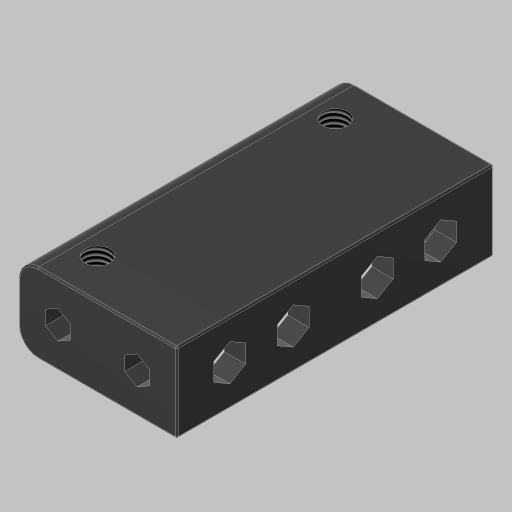
# Autodesk Inventor part: EL2-038
Saved by Autodesk Inventor 2023.5 (Build 275446000, 446)
## iProperties
Created: 2025-01-21
Part Number: EL2-038
Material: Thermoplastic Resin
Document SubType Name: Modeling
Designer: slick
Density: 1.28 g/cm^3
Appearance: Smooth - Black
Author: slick
Autodesk Inventor part; units mm, degrees
ref_plane "YZ Plane" through (0, 0, 0) normal (1, 0, 0) x (0, 1, 0)
ref_plane "XZ Plane" through (0, 0, 0) normal (0, 1, 0) x (-1, 0, 0)
ref_plane "XY Plane" through (0, 0, 0) normal (0, 0, 1) x (1, 0, 0)
sketch "Sketch1" plane through (0, 0, 0) normal (0, 0, 1) x (1, 0, 0)
  line L0 (-12.7, 6.35) -> (12.7, 6.35)
  line L1 (12.7, 6.35) -> (12.7, -6.35)
  line L2 (12.7, -6.35) -> (-12.7, -6.35)
  line L3 (-12.7, -6.35) -> (-12.7, 6.35)
  line L4 (-12.7, 6.35) -> (12.7, -6.35) construction
  line L5 (12.7, 6.35) -> (-12.7, -6.35) construction
  point P0 (0, 0)
  dimension "d0" = 25.4
  dimension "d1" = 12.7
  constraints: 12 end point, 2 midpoint, 2 parallel, 1 horizontal, 1 perpendicular
  measures "d0" distance of L1.end L2.end
  measures "d1" distance of L0.end L1.end
extrude "Extrusion1" add sketch "Sketch1" along normal mid plane 50.8
sketch "Sketch2" plane through (-12.7, 6.35, 25.4) normal (0, 1, 0) x (1, 0, 0)
  line L0 (6.35, 44.45) -> (6.35, 6.35) construction
  line L1 (0, 50.8) -> (0, 0) projected
  point P0 (12.7, 25.4)
  point P1 (6.35, 25.4)
  dimension "d4" = 38.1
  dimension "d5" = 6.35
  constraints: 2 end point, 1 horizontal alignment, 1 midpoint, 1 vertical, 1 vertical alignment
  measures "d4" distance of L0.start L0.end
  measures "d5" distance between parallel lines of L1 L0
hole "Hole1" at (-6.35, 6.35, 19.05) at (-6.35, 6.35, -19.05) direction (0, -1, 0) diameter 3.9624 end through all thread size "10-32 UNF" class "2B" standard "ANSI Unified Screw Threads"
fillet "Fillet1" radius 3.175 2 edges at (-12.7, 6.35, 0) (-12.7, -6.35, 0)
fillet "Fillet2" radius 0.254 14 edges at (-11.7701, 5.4201, 25.4) (-12.7, 0, 25.4) (-11.7701, -5.4201, 25.4) (1.5875, -6.35, 25.4) (1.5875, 6.35, 25.4) (12.7, 6.35, 0) (12.7, -6.35, 0) (12.7, 0, -25.4) (12.7, 0, 25.4) (-11.7701, 5.4201, -25.4) (-12.7, 0, -25.4) (-11.7701, -5.4201, -25.4) (1.5875, -6.35, -25.4) (1.5875, 6.35, -25.4)
sketch "Sketch3" plane through (-9.525, -6.35, 25.146) normal (0, -1, 0) x (1, 0, 0)
  line L0 (21.971, -50.292) -> (21.971, 0) projected
  line L1 (0, 0) -> (21.971, 0) projected
  line L2 (0, 0) -> (0, -50.292) projected
  line L3 (21.971, -50.292) -> (0, -50.292) projected
  circle A0 centre (3.175, -6.096) radius 1.9812 projected
  circle A1 centre (3.175, -44.196) radius 1.9812 projected
  line L4 (18.796, -3.175) -> (18.796, -47.117)
  line L5 (18.796, -47.117) -> (3.175, -47.117) construction
  line L6 (3.175, -47.117) -> (3.175, -3.175) construction
  line L7 (3.175, -3.175) -> (18.796, -3.175) construction
  circle A2 centre (3.175, -6.096) radius 5.1562 construction
  circle A3 centre (3.175, -44.196) radius 5.1562 construction
  line L8 (18.796, -3.175) -> (7.424, -3.175)
  line L9 (7.424, -47.117) -> (18.796, -47.117)
  arc A4 (0, -10.1587) -> (7.424, -3.175) centre (3.175, -6.096) ccw
  circle A5 centre (3.175, -44.196) radius 1.9812 projected
  arc A6 (7.424, -47.117) -> (0, -40.1333) centre (3.175, -44.196) ccw
  line L10 (21.971, -50.292) -> (21.971, 0) construction
  line L11 (0, 0) -> (21.971, 0) construction
  line L12 (0, 0) -> (0, -50.292) construction
  line L13 (21.971, -50.292) -> (0, -50.292) construction
  circle A7 centre (3.175, -6.096) radius 1.9812 construction
  circle A8 centre (3.175, -44.196) radius 1.9812 construction
  line L14 (0, 0) -> (0, -50.292) projected
  line L15 (0, -40.1333) -> (0, -10.1587)
  point P0 (9.525, -25.146)
  dimension "d15" = 3.175
  dimension "d16" = 3.175
  dimension "d17" = 3.175
  constraints: 14 end point, 8 point on circle, 4 centre point, 4 point on line, 2 coincident, 3 other
  measures "d15" distance between parallel lines of L0 L4
  measures "d16" radial gap between concentric circles of A0 A2
  measures "d17" radial gap between concentric circles of A1 A3
extrude "Extrusion2" cut sketch "Sketch3" against normal blind 9.525 contours L2 A4 L8 L4 L9 A6
fillet "Fillet3" radius 3.302 6 edges at (-2.101, -1.5875, 21.971) (9.271, -1.5875, 21.971) (9.271, -1.5875, -21.971) (-2.101, -1.5875, -21.971) (-9.525, -1.5875, -14.9873) (-9.525, -1.5875, 14.9873)
sketch "Sketch4" plane through (12.7, -6.096, 25.146) normal (1, 0, 0) x (0, 0, -1)
  line L0 (8.255, 9.0289) -> (10.795, 7.5625)
  line L1 (10.795, 7.5625) -> (10.795, 4.6295)
  line L2 (10.795, 4.6295) -> (8.255, 3.1631)
  line L3 (8.255, 3.1631) -> (5.715, 4.6295)
  line L4 (5.715, 4.6295) -> (5.715, 7.5625)
  line L5 (5.715, 7.5625) -> (8.255, 9.0289)
  line L6 (0, 0) -> (0, 12.192) construction
  line L7 (0, 12.192) -> (50.292, 12.192) construction
  line L8 (18.415, 9.0289) -> (20.955, 7.5625)
  line L9 (20.955, 7.5625) -> (20.955, 4.6295)
  line L10 (20.955, 4.6295) -> (18.415, 3.1631)
  line L11 (18.415, 3.1631) -> (15.875, 4.6295)
  line L12 (15.875, 4.6295) -> (15.875, 7.5625)
  line L13 (15.875, 7.5625) -> (18.415, 9.0289)
  line L14 (25.146, 12.192) -> (25.146, -0.254) construction
  line L15 (0, -0.254) -> (50.292, -0.254) construction
  line L16 (42.037, 9.0289) -> (39.497, 7.5625)
  line L17 (39.497, 7.5625) -> (39.497, 4.6295)
  line L18 (39.497, 4.6295) -> (42.037, 3.1631)
  line L19 (42.037, 3.1631) -> (44.577, 4.6295)
  line L20 (44.577, 4.6295) -> (44.577, 7.5625)
  line L21 (44.577, 7.5625) -> (42.037, 9.0289)
  line L22 (31.877, 9.0289) -> (29.337, 7.5625)
  line L23 (29.337, 7.5625) -> (29.337, 4.6295)
  line L24 (29.337, 4.6295) -> (31.877, 3.1631)
  line L25 (31.877, 3.1631) -> (34.417, 4.6295)
  line L26 (34.417, 4.6295) -> (34.417, 7.5625)
  line L27 (34.417, 7.5625) -> (31.877, 9.0289)
  point P0 (25.146, 6.096)
  point P1 (8.255, 6.096)
  point P2 (10.795, 6.096)
  point P3 (5.715, 6.096)
  point P4 (18.415, 6.096)
  point P5 (20.955, 6.096)
  point P6 (15.875, 6.096)
  point P7 (42.037, 6.096)
  point P8 (39.497, 6.096)
  point P9 (44.577, 6.096)
  point P10 (31.877, 6.096)
  point P11 (29.337, 6.096)
  point P12 (34.417, 6.096)
  dimension "d21" = 5.08
  dimension "d25" = 10.16
  dimension "d35" = 6.731
  constraints: 50 end point, 18 symmetric about line, 4 midpoint, 1 horizontal, 1 horizontal alignment, 1 vertical, 28 other
  measures "d21" distance of point (10.795, 6.096) point (5.715, 6.096)
  measures "d25" distance of point (8.255, 6.096) point (18.415, 6.096)
  measures "d35" distance from line of L14 point (18.415, 6.096)
extrude "Extrusion3" cut sketch "Sketch4" against normal through all
sketch "Sketch5" plane through (0, 0, 25.4) normal (0, 0, 1) x (1, 0, 0)
  line L0 (-4.3688, -6.35) -> (-4.3688, 6.35) construction
  line L1 (-4.3688, 1.1438) -> (-4.3688, -1.1438)
  line L2 (-4.3688, -1.1438) -> (-6.35, -2.2877)
  line L3 (-6.35, -2.2877) -> (-8.3312, -1.1438)
  line L4 (-8.3312, -1.1438) -> (-8.3312, 1.1438)
  line L5 (-8.3312, 1.1438) -> (-6.35, 2.2877)
  line L6 (-6.35, 2.2877) -> (-4.3688, 1.1438)
  line L7 (0, 6.096) -> (0, -7.4763) construction
  line L8 (-9.525, 6.096) -> (12.446, 6.096) construction
  line L9 (4.3688, 1.1438) -> (4.3688, -1.1438)
  line L10 (4.3688, -1.1438) -> (6.35, -2.2877)
  line L11 (6.35, -2.2877) -> (8.3312, -1.1438)
  line L12 (8.3312, -1.1438) -> (8.3312, 1.1438)
  line L13 (8.3312, 1.1438) -> (6.35, 2.2877)
  line L14 (6.35, 2.2877) -> (4.3688, 1.1438)
  point P0 (0, 0)
  point P1 (-6.35, 0)
  point P2 (0, -0.6901)
  point P3 (6.35, 0)
  dimension "d32" = 6.35
  constraints: 26 end point, 7 symmetric about line, 2 point on line, 2 vertical, 1 horizontal alignment, 1 midpoint, 1 vertical alignment, 13 other
  measures "d32" distance from line of L7 point (-6.35, 0)
extrude "Extrusion4" cut sketch "Sketch5" against normal through all
body "Solid1"
